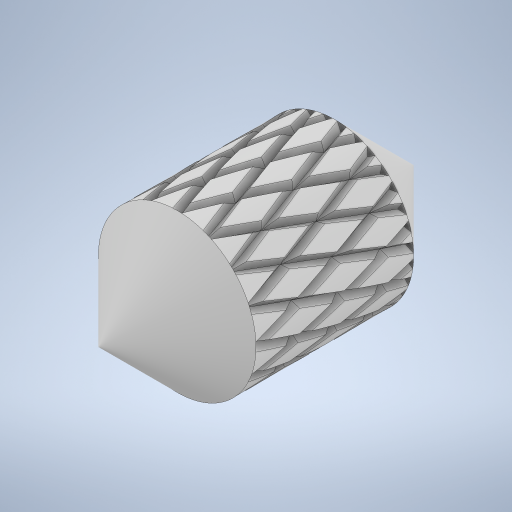
# Autodesk Inventor part: Pino Recartilhado Tangencial
Saved by Autodesk Inventor 2023 (Build 270158030, 158C)
## iProperties
Created: 2022-07-26
Part Number: Pino Recartilhado Tangencial
Material: Generic
Document SubType Name: Modeling
Designer: coqui
Density: 1 g/cm^3
Appearance: Default
Author: coqui
Autodesk Inventor part; units mm, degrees
ref_plane "YZ Plane" through (0, 0, 0) normal (1, 0, 0) x (0, 1, 0)
ref_plane "XZ Plane" through (0, 0, 0) normal (0, 1, 0) x (-1, 0, 0)
sketch "Sketch1" plane through (0, 0, 0) normal (0, 0, 1) x (1, 0, 0)
  circle A0 centre (0, 0) radius 10
  dimension "d0" = 20
  constraints: 1 centre point, 1 coincident
  measures "d0" diameter of A0
extrude "Extrusion1" add sketch "Sketch1" along normal mid plane 40
ref_plane "Work Plane1" through (0, 0, 10) normal (0, 0, 1) x (1, 0, 0)
sketch "Sketch2" plane through (0, 0, 10) normal (0, 0, 1) x (1, 0, 0)
  line L0 (0, 9) -> (-0.866, 10.5)
  line L1 (-0.866, 10.5) -> (0.866, 10.5)
  line L2 (0.866, 10.5) -> (0, 9)
  point P0 (0, 0)
  point P1 (0, 10)
  dimension "d4" = 10
  dimension "d5" = 1
  constraints: 6 end point, 7 other
  measures "d4" distance of point (0, 0) point (0, 10)
  measures "d5" distance of L0.start point (0, 10)
sketch "Sketch3" plane through (0, 0, 0) normal (0, 1, 0) x (-1, 0, 0)
  line L0 (0, 9.9624) -> (0, -26.8928) construction
  point P0 (0, 0)
  constraints: 2 end point, 1 vertical
coil "Coil1" sketch "Sketch2" operation cut axis through (0, 0, 9.9624) along (0, 0, -1) pitch 180 turns 0.111111 hand right
mirror "Mirror2" about plane through (0, 0, 0) normal (1, 0, 0) of "Coil1"
pattern_circular "Circular Pattern1" count 16 over 360 about axis through (0, 0, 0) along (0, 0, 1) of "Coil1", "Mirror2"
chamfer "Chamfer1" distance 10 angle 45 2 edges at (-10, 0, 20) (-10, 0, -20)
body "Solid1"
